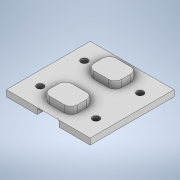
# Autodesk Inventor part: sensorbar
Saved by Autodesk Inventor 2022 (Build 260153000, 153)
## iProperties
Created: 2023-02-05
Part Number: sensorbar
Material: 一般
Document SubType Name: Modeling
Designer: Yazawa
Density: 1 g/cm^3
Appearance: 既定
Author: Yazawa
Autodesk Inventor part; units mm, degrees
ref_plane "YZ Plane" through (0, 0, 0) normal (1, 0, 0) x (0, 1, 0)
ref_plane "XZ Plane" through (0, 0, 0) normal (0, 1, 0) x (-1, 0, 0)
ref_plane "XY Plane" through (0, 0, 0) normal (0, 0, 1) x (1, 0, 0)
sketch "スケッチ1" plane through (0, 0, 0) normal (0, 1, 0) x (-1, 0, 0)
  line L0 (9.5, -9.5) -> (0, -9.5)
  line L1 (0, -9.5) -> (0, -2.5)
  line L2 (0, 0) -> (3.15, 0)
  line L3 (9.5, 0) -> (9.5, -9.5)
  line L4 (0, 0) -> (3.15, 0)
  line L5 (3.15, 0) -> (3.15, -1)
  line L6 (1.65, -2.5) -> (0, -2.5)
  line L7 (0, -2.5) -> (0, 0)
  arc A0 (1.65, -2.5) -> (3.15, -1) centre (1.65, -1) ccw
  line L8 (3.15, 0) -> (6.325, 0)
  line L9 (6.325, 0) -> (9.5, 0)
  line L10 (0, -2.5) -> (0, 0)
  line L11 (9.5, 9.5) -> (0, 9.5)
  line L12 (9.5, 0) -> (9.5, 9.5)
  line L13 (3.15, 0) -> (3.15, 1)
  line L14 (1.65, 2.5) -> (0, 2.5)
  arc A1 (3.15, 1) -> (1.65, 2.5) centre (1.65, 1) ccw
  line L15 (-9.5, -9.5) -> (0, -9.5)
  line L16 (-9.5, 0) -> (-9.5, -9.5)
  line L17 (-3.15, 0) -> (-3.15, -1)
  line L18 (-1.65, -2.5) -> (0, -2.5)
  arc A2 (-3.15, -1) -> (-1.65, -2.5) centre (-1.65, -1) ccw
  line L19 (-9.5, 9.5) -> (0, 9.5)
  line L20 (-9.5, 0) -> (-9.5, 9.5)
  line L21 (-3.15, 0) -> (-3.15, 1)
  arc A3 (-1.65, 2.5) -> (-3.15, 1) centre (-1.65, 1) ccw
  line L22 (-1.65, 2.5) -> (0, 2.5)
  point P0 (-6.325, 0)
  dimension "d2" = 1.5
  dimension "d3" = 19
  dimension "d4" = 6.3
  dimension "d5" = 5
  dimension "d6" = 19
  constraints: 46 end point, 17 symmetric about line, 8 point on circle, 5 parallel, 4 centre point, 3 horizontal, 3 perpendicular, 2 coincident, 2 collinear, 2 tangent, 3 other
  measures "d2" radius of A0
  measures "d3" distance between parallel lines of L16 L3
  measures "d4" distance between parallel lines of L17 L5
  measures "d5" distance between parallel lines of L14 L6
  measures "d6" distance between parallel lines of L11 L0
extrude "押し出し1" add sketch "スケッチ1" along normal blind 1.4
sketch "スケッチ2" plane through (0, 1.4, 0) normal (0, 1, 0) x (1, 0, 0)
  line L0 (9.5, 9.5) -> (-9.5, 9.5) projected
  line L1 (0, 9.5) -> (0, 7.5)
  line L2 (0, 7.5) -> (0, 2.5)
  line L3 (0, 2.5) -> (0, 0)
  line L4 (-3.15, 7.5) -> (3.15, 7.5)
  line L5 (3.15, 7.5) -> (3.15, 2.5)
  line L6 (3.15, 2.5) -> (-3.15, 2.5)
  line L7 (-3.15, 2.5) -> (-3.15, 7.5)
  line L8 (-9.5, 9.5) -> (-9.5, -9.5) projected
  line L9 (-9.5, 0) -> (9.5, 0)
  line L10 (9.5, -9.5) -> (9.5, 9.5) projected
  line L11 (-3.15, -7.5) -> (3.15, -7.5)
  line L12 (3.15, -7.5) -> (3.15, -2.5)
  line L13 (3.15, -2.5) -> (-3.15, -2.5)
  line L14 (-3.15, -2.5) -> (-3.15, -7.5)
  dimension "d11" = 6.3
  dimension "d12" = 2.5
  dimension "d13" = 5
  constraints: 24 end point, 6 midpoint, 4 symmetric about line, 3 coincident, 2 parallel, 2 point on line, 1 horizontal, 1 perpendicular, 1 vertical
  measures "d11" distance between parallel lines of L5 L7
  measures "d12" distance of L2.end L3.end
  measures "d13" distance of L4.end L5.end
extrude "押し出し2" add sketch "スケッチ2" along normal blind 1.6 contours L4 L5 L6 L2 | L2 L6 L7 L4 | L14 L13 L12 L11
fillet "フィレット1" radius 1.5 8 edges at (-3.15, 2.2, -2.5) (-3.15, 2.2, 7.5) (3.15, 2.2, 7.5) (3.15, 2.2, 2.5) (-3.15, 2.2, 2.5) (3.15, 2.2, -2.5) (3.15, 2.2, -7.5) (-3.15, 2.2, -7.5)
sketch "スケッチ3" plane through (0, 1.4, 0) normal (0, 1, 0) x (1, 0, 0)
  arc A0 (-1.65, 7.5) -> (-3.15, 6) centre (-1.65, 6) ccw projected
  line L0 (-3.15, 6) -> (-3.15, 4) projected
  arc A1 (-3.15, 4) -> (-1.65, 2.5) centre (-1.65, 4) ccw projected
  line L1 (-1.65, 2.5) -> (1.65, 2.5) projected
  arc A2 (1.65, 2.5) -> (3.15, 4) centre (1.65, 4) ccw projected
  line L2 (3.15, 4) -> (3.15, 6) projected
  arc A3 (3.15, 6) -> (1.65, 7.5) centre (1.65, 6) ccw projected
  line L3 (1.65, 7.5) -> (-1.65, 7.5) projected
  arc A4 (-1.65, -2.5) -> (-3.15, -4) centre (-1.65, -4) ccw projected
  line L4 (-3.15, -4) -> (-3.15, -6) projected
  arc A5 (-3.15, -6) -> (-1.65, -7.5) centre (-1.65, -6) ccw projected
  line L5 (-1.65, -7.5) -> (1.65, -7.5) projected
  arc A6 (1.65, -7.5) -> (3.15, -6) centre (1.65, -6) ccw projected
  line L6 (3.15, -6) -> (3.15, -4) projected
  arc A7 (3.15, -4) -> (1.65, -2.5) centre (1.65, -4) ccw projected
  line L7 (1.65, -2.5) -> (-1.65, -2.5) projected
  line L8 (-3.15, 5) -> (-9.5, 5)
  line L9 (-9.5, 9.5) -> (-9.5, -9.5) projected
  line L10 (-9.5, 0) -> (0, 0)
  line L11 (0, 0) -> (0, 9.5)
  line L12 (9.5, 9.5) -> (-9.5, 9.5) projected
  point P0 (-6.325, 5)
  point P1 (-6.325, -5)
  point P2 (6.325, 5)
  point P3 (6.325, -5)
  constraints: 6 end point, 4 midpoint, 3 symmetric about line, 2 horizontal, 1 point on line
hole "穴1" at (-6.325, 1.4, -5) at (-6.325, 1.4, 5) at (6.325, 1.4, -5) at (6.325, 1.4, 5) direction (0, -1, 0) diameter 1.567 end through all thread size "M2x0.4" class "6H" standard "ISO Metric profile"
sketch "スケッチ4" plane through (0, 0, 0) normal (0, -1, 0) x (1, 0, 0)
  line L0 (-2.5, 9.5) -> (2.5, 9.5)
  line L1 (2.5, 9.5) -> (2.5, 6.5)
  line L2 (2.5, 6.5) -> (-2.5, 6.5)
  line L3 (-2.5, 6.5) -> (-2.5, 9.5)
  line L4 (-9.5, 9.5) -> (9.5, 9.5) projected
  point P0 (0, 0)
  point P1 (0, 9.5)
  dimension "d24" = 5
  dimension "d25" = 3
  constraints: 8 end point, 2 midpoint, 2 parallel, 1 collinear, 1 horizontal, 1 perpendicular
  measures "d24" distance of L1.end L2.end
  measures "d25" distance of L0.end L1.end
extrude "押し出し3" cut sketch "スケッチ4" against normal blind 1.6
sketch "スケッチ5" plane through (-2.5, 0, 9.5) normal (1, 0, 0) x (0, 0, -1)
  line L0 (2.2641, 1.4) -> (2.2641, 1.6) projected
  line L1 (0, 1.4) -> (2.2641, 1.4) projected
  line L2 (0, 0) -> (0, 1.4) projected
  line L3 (3, 0) -> (0, 0) projected
  line L4 (3, 0) -> (3, 1.6) projected
  line L5 (3, 1.6) -> (2.2641, 1.6) projected
  spline S0 degree 2 poles (3, 0) (2.1867, 1.089) (0, 1.4) knots 0 0 0 1 1 1
  point P0 (9.5, 0)
  point P1 (2.0329, 0.8)
  constraints: 3 other
extrude "押し出し4" add sketch "スケッチ5" along normal up to surface (5 mm away) contours L0 L5 L4 S0 L1
sketch "スケッチ6" plane through (0, 1.6, 0) normal (0, -1, 0) x (1, 0, 0)
  line L0 (-2.5, 7.2359) -> (2.5, 7.2359) projected
  arc A0 (2.5, 7.2359) -> (1.65, 7.5) centre (1.65, 6) ccw projected
  line L1 (-1.65, 7.5) -> (1.65, 7.5) projected
  arc A1 (-1.65, 7.5) -> (-2.5, 7.2359) centre (-1.65, 6) ccw projected
  point P0 (0, 0)
extrude "押し出し5" add sketch "スケッチ6" along normal up to surface (0.2 mm away)
fillet "フィレット2" radius 0.5 2 edges at (-2.5, 0.8945, 7.6566) (2.5, 0.8945, 7.6566)
